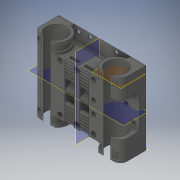
# Autodesk Inventor part: X-Carriage_back
Saved by Autodesk Inventor 2019 (Build 230136000, 136)
## iProperties
Created: 2019-09-14
Part Number: X-Carriage_back
Material: ABS-Kunststoff
Document SubType Name: Modeling
Designer: marc
Density: 1.06 g/cm^3
Appearance: Grau
Author: marc
## iProperties of the stored document X-Carriage_back_3D-Druck.ipt
Created: 2019-09-14
Part Number: X-Carriage_back_3D-Druck
Material: Generisch
Document SubType Name: Modeling
Designer: marc
Density: 1 g/cm^3
Appearance: Vorgabe
Author: marc
Autodesk Inventor part; units mm, degrees
ref_plane "YZ Plane" through (0, 0, 0) normal (1, 0, 0) x (0, 1, 0)
ref_plane "XZ Plane" through (0, 0, 0) normal (0, 1, 0) x (-1, 0, 0)
ref_plane "XY Plane" through (0, 0, 0) normal (0, 0, 1) x (1, 0, 0)
sketch "Skizze1" plane through (0, 0, 0) normal (0, 1, 0) x (-1, 0, 0)
  line L0 (0, 0) -> (65, 0)
  line L1 (65, 0) -> (65, 21.4)
  line L2 (65, 21.4) -> (0, 21.4)
  line L3 (0, 21.4) -> (0, 0)
  dimension "d0" = 65
  dimension "d1" = 21.4
  constraints: 8 end point, 2 parallel, 1 horizontal, 1 perpendicular
  measures "d0" distance of L2.end L1.end
  measures "d1" distance of L1.end L0.end
extrude "Extrusion1" add sketch "Skizze1" along normal blind 55
sketch "Skizze2" plane through (0, 0, 0) normal (0, -1, 0) x (1, 0, 0)
  line L0 (-65, 0) -> (-65, 21.4) projected
  line L1 (-65, 21.4) -> (0, 21.4) projected
  point P0 (0, 0)
  point P1 (-55, 9.4)
  point P2 (-10, 9.4)
  dimension "d4" = 10
  dimension "d5" = 45
  dimension "d6" = 12
  constraints: 1 horizontal alignment
  measures "d4" distance from line of L0 point (-55, 9.4)
  measures "d5" distance of point (-55, 9.4) point (-10, 9.4)
  measures "d6" distance from line of L1 point (-55, 9.4)
hole "Bohrung1" at (-55, 0, 9.4) at (-10, 0, 9.4) direction (0, 1, 0) diameter 15 end through all
sketch "Skizze7" plane through (0, 55, 0) normal (0, 1, 0) x (1, 0, 0)
  line L0 (-65, 0) -> (-65, -21.4) projected
  line L1 (0, -21.4) -> (0, 0) projected
  line L2 (-65, -21.4) -> (0, -21.4)
  line L3 (0, -21.4) -> (0, -16.4)
  line L4 (0, -16.4) -> (-65, -16.4)
  line L5 (-65, -16.4) -> (-65, -21.4)
  dimension "d49" = 5
  constraints: 8 end point, 2 parallel, 1 horizontal, 1 perpendicular, 1 point on line
  measures "d49" distance between parallel lines of L2 L4
extrude "Extrusion5" cut sketch "Skizze7" against normal up to next
sketch "Skizze8" plane through (0, 55, 0) normal (0, 1, 0) x (1, 0, 0)
  arc A0 (-52.3074, -16.4) -> (-57.6926, -16.4) centre (-55, -9.4) ccw projected
  line L0 (-45.7129, -11.4) -> (-19.2871, -11.4)
  arc A1 (-7.3074, -16.4) -> (-12.6926, -16.4) centre (-10, -9.4) ccw projected
  line L1 (0, 0) -> (-65, 0) projected
  line L2 (-52.3074, -16.4) -> (-12.6926, -16.4) projected
  arc A2 (-48.5774, -16.4) -> (-45.7129, -11.4) centre (-55, -9.4) ccw
  arc A3 (-19.2871, -11.4) -> (-16.4226, -16.4) centre (-10, -9.4) ccw
  dimension "d52" = 11.4
  dimension "d55" = 9.5
  dimension "d56" = 9.5
  constraints: 4 point on circle, 2 centre point, 2 coincident, 2 end point, 2 point on line, 1 horizontal
  measures "d52" distance between parallel lines of L1 L0
  measures "d55" radius of A3
  measures "d56" radius of A2
extrude "Extrusion6" cut sketch "Skizze8" against normal blind 7
ref_plane "Arbeitsebene3" through (0, 27.5, 0) normal (0, -1, 0) x (1, 0, 0)
mirror "Spiegeln3" about plane through (0, 27.5, 0) normal (0, -1, 0) of "Extrusion6"
ref_plane "Arbeitsebene4" through (-32.5, 0, 0) normal (-1, 0, 0) x (0, 0, 1)
sketch "Skizze9" plane through (0, 48, 0) normal (0, 1, 0) x (1, 0, 0)
  line L0 (-45.7129, -11.4) -> (-19.2871, -11.4) projected
  line L1 (-34.5, -11.4) -> (-41.5, -11.4)
  line L2 (-41.5, -11.4) -> (-41.5, -13.4)
  line L3 (-41.5, -13.4) -> (-34.5, -13.4)
  line L4 (-34.5, -13.4) -> (-34.5, -11.4)
  line L5 (-32.5, -19.68) -> (-32.5, 3.28) projected
  point P0 (0, 0)
  dimension "d59" = 7
  dimension "d60" = 2
  dimension "d61" = 2
  constraints: 8 end point, 2 parallel, 1 horizontal, 1 perpendicular, 1 point on line
  measures "d59" distance of L3.end L2.end
  measures "d60" distance of L2.end L1.end
  measures "d61" distance between parallel lines of L5 L4
extrude "Extrusion7" cut sketch "Skizze9" against normal blind 20
mirror "Spiegeln4" about plane through (-32.5, 0, 0) normal (-1, 0, 0) of "Extrusion7"
mirror "Spiegeln5" about plane through (0, 27.5, 0) normal (0, -1, 0) of "Extrusion7", "Spiegeln4"
sketch "Skizze10" plane through (-12.6926, 0, 16.4) normal (0, 0, 1) x (1, 0, 0)
  line L0 (-28.8074, 7) -> (-28.8074, 27) projected
  line L1 (-10.8074, 27) -> (-17.8074, 27) projected
  line L2 (-10.8074, 7) -> (-10.8074, 27) projected
  line L3 (-17.8074, 27) -> (-10.8074, 27)
  line L4 (-10.8074, 27) -> (-10.8074, 20)
  line L5 (-17.8074, 48) -> (-17.8074, 28) projected
  line L6 (-10.8074, 48) -> (-10.8074, 28) projected
  line L7 (-17.8074, 28) -> (-10.8074, 28)
  line L8 (-10.8074, 28) -> (-10.8074, 35)
  line L9 (-10.8074, 35) -> (-17.8074, 35)
  line L10 (-17.8074, 35) -> (-17.8074, 28)
  line L11 (-21.8074, 48) -> (-21.8074, 28) projected
  line L12 (-21.8074, 28) -> (-28.8074, 28)
  line L13 (-28.8074, 28) -> (-28.8074, 35)
  line L14 (-28.8074, 35) -> (-21.8074, 35)
  line L15 (-21.8074, 35) -> (-21.8074, 28)
  line L16 (-10.8074, 20) -> (-17.8074, 20)
  line L17 (-17.8074, 7) -> (-17.8074, 27) projected
  line L18 (-17.8074, 20) -> (-17.8074, 27)
  line L19 (-21.8074, 7) -> (-21.8074, 27) projected
  line L20 (-28.8074, 7) -> (-28.8074, 27) projected
  line L21 (-21.8074, 27) -> (-28.8074, 27)
  line L22 (-28.8074, 27) -> (-28.8074, 20)
  line L23 (-28.8074, 20) -> (-21.8074, 20)
  line L24 (-21.8074, 20) -> (-21.8074, 27)
  point P0 (12.6926, 0)
  dimension "d67" = 7
  dimension "d68" = 7
  dimension "d69" = 7
  constraints: 32 end point, 7 parallel, 7 point on line, 5 horizontal, 4 perpendicular, 1 vertical alignment
  measures "d67" distance between parallel lines of L7 L9
  measures "d68" distance of L3.end L4.end
  measures "d69" distance between parallel lines of L21 L23
extrude "Extrusion8" cut sketch "Skizze10" against normal up to next
fillet "Rundung3" radius 7 4 edges at (-38, 28, 11.4) (-27, 28, 11.4) (-38, 27, 11.4) (-27, 27, 11.4)
fillet "Rundung4" radius 1.5 8 edges at (-38, 35, 16.4) (-38, 35, 13.4) (-27, 35, 16.4) (-27, 35, 13.4) (-38, 20, 13.4) (-38, 20, 16.4) (-27, 20, 13.4) (-27, 20, 16.4)
sketch "Skizze11" plane through (-12.6926, 0, 16.4) normal (0, 0, 1) x (1, 0, 0)
  line L0 (-19.8074, -11) -> (-19.8074, 66) projected
  line L1 (-35.8848, 7) -> (-3.73, 7) projected
  point P0 (12.6926, 0)
  point P1 (-32.3074, 10)
  point P2 (-19.8074, 10)
  point P3 (-7.3074, 10)
  dimension "d71" = 12.5
  dimension "d72" = 12.5
  dimension "d73" = 3
  constraints: 2 horizontal alignment, 1 point on line
  measures "d71" distance from line of L0 point (-7.307, 10)
  measures "d72" distance from line of L0 point (-32.307, 10)
  measures "d73" distance from line of L1 point (-32.307, 10)
hole "Bohrung2" at (-45, 10, 16.4) at (-32.5, 10, 16.4) at (-20, 10, 16.4) direction (0, 0, -1) diameter 3.75 depth 8 tip angle 118
mirror "Spiegeln6" about plane through (0, 27.5, 0) normal (0, -1, 0) of "Bohrung2"
sketch "Skizze15" plane through (-12.6926, 0, 16.4) normal (0, 0, 1) x (1, 0, 0)
  line L0 (-28.8074, 7) -> (-21.8074, 7)
  line L1 (-21.8074, 7) -> (-21.8074, 18.5)
  line L2 (-21.8074, 18.5) -> (-28.8074, 18.5)
  line L3 (-28.8074, 18.5) -> (-28.8074, 7)
  line L4 (-35.8848, 7) -> (-3.73, 7) projected
  circle A0 centre (-32.3074, 10) radius 1.875 projected
  line L5 (-19.8074, -11) -> (-19.8074, 66) projected
  line L6 (-17.8074, 7) -> (-10.8074, 7)
  line L7 (-10.8074, 7) -> (-10.8074, 18.5)
  line L8 (-10.8074, 18.5) -> (-17.8074, 18.5)
  line L9 (-17.8074, 18.5) -> (-17.8074, 7)
  point P0 (12.6926, 0)
  constraints: 16 end point, 6 coincident, 4 parallel, 2 horizontal, 2 perpendicular, 2 point on line
extrude "Extrusion10" cut sketch "Skizze15" against normal blind 1.4 contours L3 L2 L1 L0 | L9 L8 L7 L4
sketch "Skizze16" plane through (-30.5, 7, 16.4) normal (1, 0, 0) x (0, 0, -1)
  line L0 (0, 0) -> (0, 11.5) projected
  line L1 (0, 11.5) -> (1.4, 11.5) projected
  line L2 (1.4, 0) -> (1.4, 11.5) projected
  line L3 (1.4, 0) -> (0, 0) projected
  arc A0 (0, 11.5) -> (0.4324, 10.9587) centre (0.555, 11.5) ccw
  arc A1 (0.4324, 10.9587) -> (1.024, 10.9328) centre (0.77, 11.9) ccw
  arc A2 (0.4324, 2.0413) -> (0.4324, 0.9587) centre (0.555, 1.5) ccw
  arc A3 (0.4324, 4.0413) -> (0.4324, 2.9587) centre (0.555, 3.5) ccw
  arc A4 (0.4324, 6.0413) -> (0.4324, 4.9587) centre (0.555, 5.5) ccw
  arc A5 (0.4324, 8.0413) -> (0.4324, 6.9587) centre (0.555, 7.5) ccw
  arc A6 (0.4324, 10.0413) -> (0.4324, 8.9587) centre (0.555, 9.5) ccw
  arc A7 (0.4324, 8.9587) -> (1.024, 8.9328) centre (0.77, 9.9) ccw
  arc A8 (1.024, 10.0672) -> (0.4324, 10.0413) centre (0.77, 9.1) ccw
  arc A9 (1.024, 8.0672) -> (0.4324, 8.0413) centre (0.77, 7.1) ccw
  arc A10 (0.4324, 6.9587) -> (1.024, 6.9328) centre (0.77, 7.9) ccw
  arc A11 (1.024, 2.0672) -> (0.4324, 2.0413) centre (0.77, 1.1) ccw
  arc A12 (0.4324, 4.9587) -> (1.024, 4.9328) centre (0.77, 5.9) ccw
  line L4 (1.024, 10.0672) -> (1.024, 10.9328)
  line L5 (1.024, 8.0672) -> (1.024, 8.9328)
  arc A13 (1.024, 6.0672) -> (0.4324, 6.0413) centre (0.77, 5.1) ccw
  line L6 (1.024, 6.0672) -> (1.024, 6.9328)
  line L7 (1.024, 4.0672) -> (1.024, 4.9328)
  line L8 (1.024, 0) -> (1.024, 0.9328)
  line L9 (1.024, 2.0672) -> (1.024, 2.9328)
  arc A14 (1.024, 4.0672) -> (0.4324, 4.0413) centre (0.77, 3.1) ccw
  arc A15 (0.4324, 2.9587) -> (1.024, 2.9328) centre (0.77, 3.9) ccw
  arc A16 (0.4324, 0.9587) -> (1.024, 0.9328) centre (0.77, 1.9) ccw
  point P0 (16.4, -7)
  point P1 (0.77, 11.1)
  dimension "d97" = 0.555
  dimension "d101" = 2
  dimension "d103" = 0.63
  dimension "d104" = 0.4
  dimension "d106" = 2
  dimension "d107" = 2
  dimension "d108" = 2
  dimension "d109" = 2
  dimension "d112" = 0.4
  dimension "d115" = 0.4
  dimension "d116" = 0.4
  dimension "d117" = 0.4
  dimension "d118" = 0.4
  dimension "d119" = 0.4
  dimension "d120" = 0.4
  dimension "d121" = 0.4
  dimension "d151" = 2
  dimension "d152" = 0.4
  dimension "d166" = 0.376
  dimension "d167" = 0.376
  dimension "d168" = 0.376
  dimension "d169" = 0.376
  dimension "d170" = 0.376
  dimension "d171" = 1
  dimension "d172" = 1
  dimension "d173" = 0.555
  dimension "d174" = 1
  dimension "d175" = 1
  dimension "d176" = 1
  dimension "d177" = 1
  dimension "d178" = 1
  dimension "d179" = 1
  dimension "d180" = 1
  dimension "d181" = 1
  dimension "d182" = 0.4
  dimension "d183" = 0.4
  dimension "d184" = 0.376
  constraints: 34 point on circle, 17 centre point, 16 coincident, 16 vertical alignment, 13 end point, 6 perpendicular, 6 tangent, 3 point on line
  measures "d97" distance from line of L0 point (0.555, 11.5)
  measures "d101" distance of point (0.555, 11.5) point (0.555, 9.5)
  measures "d103" distance from line of L2 point (0.77, 11.1)
  measures "d104" distance from line of L1 point (0.77, 11.1)
  measures "d106" distance of point (0.555, 9.5) point (0.555, 7.5)
  measures "d107" distance of point (0.555, 5.5) point (0.555, 7.5)
  measures "d108" distance of point (0.555, 3.5) point (0.555, 5.5)
  measures "d109" distance of point (0.555, 1.5) point (0.555, 3.5)
  measures "d112" vertical distance of point (0.555, 9.5) point (0.77, 9.9)
  measures "d115" vertical distance of point (0.555, 7.5) point (0.77, 7.1)
  measures "d116" vertical distance of point (0.555, 5.5) point (0.77, 5.9)
  measures "d117" vertical distance of point (0.555, 5.5) point (0.77, 5.1)
  measures "d118" vertical distance of point (0.555, 3.5) point (0.77, 3.9)
  measures "d119" vertical distance of point (0.555, 3.5) point (0.77, 3.1)
  measures "d120" vertical distance of point (0.555, 1.5) point (0.77, 1.9)
  measures "d121" vertical distance of point (0.555, 1.5) point (0.77, 1.1)
  measures "d151" diameter of A1
  measures "d152" distance from line of L1 A1.centre
  measures "d166" distance between parallel lines of L2 L5
  measures "d167" distance between parallel lines of L2 L6
  measures "d168" distance between parallel lines of L2 L7
  measures "d169" distance between parallel lines of L9 L2
  measures "d170" distance between parallel lines of L8 L2
  measures "d171" radius of A11
  measures "d172" radius of A16
  measures "d173" radius of A2
  measures "d174" radius of A15
  measures "d175" radius of A14
  measures "d176" radius of A12
  measures "d177" radius of A13
  measures "d178" radius of A10
  measures "d179" radius of A9
  measures "d180" radius of A7
  measures "d181" radius of A8
  measures "d182" vertical distance of point (0.555, 9.5) point (0.77, 9.1)
  measures "d183" vertical distance of point (0.555, 7.5) point (0.77, 7.9)
  measures "d184" distance between parallel lines of L2 L4
extrude "Extrusion11" add sketch "Skizze16" along normal up to next contours A2 A11 L9 A15 A3 A14 L7 A12 A4 A13 L6 A10 A5 A9 L5 A7 A6 A8 L4 A1 A0 L1 L2 L3 L8 A16
mirror "Spiegeln7" about plane through (-32.5, 0, 0) normal (-1, 0, 0) of "Extrusion11"
mirror "Spiegeln8" about plane through (0, 27.5, 0) normal (0, -1, 0) of "Extrusion11", "Spiegeln7", "Extrusion10"
sketch "Skizze18" plane through (0, 55, 0) normal (0, 1, 0) x (1, 0, 0)
  arc A0 (-52.3074, -16.4) -> (-57.6926, -16.4) centre (-55, -9.4) ccw projected
  arc A1 (-7.3074, -16.4) -> (-12.6926, -16.4) centre (-10, -9.4) ccw projected
  line L0 (-45.7129, -11.4) -> (-41.5, -11.4) projected
  arc A2 (-45.7129, -11.4) -> (-53.6252, 0) centre (-55, -9.4) ccw
  arc A3 (-11.3748, 0) -> (-19.2871, -11.4) centre (-10, -9.4) ccw
  line L1 (-19.2871, -11.4) -> (-45.7129, -11.4) projected
  line L2 (-45.7129, -11.4) -> (-19.2871, -11.4)
  line L3 (0, 0) -> (-65, 0) projected
  line L4 (-53.6252, 0) -> (-11.3748, 0)
  dimension "d190" = 45
  dimension "d192" = 19
  constraints: 4 end point, 4 point on circle, 3 point on line, 2 centre point, 2 coincident, 1 collinear
  measures "d190" distance of A0.centre A1.centre
  measures "d192" diameter of A3
extrude "Extrusion12" cut sketch "Skizze18" against normal up to surface (7 mm away)
mirror "Spiegeln9" about plane through (0, 27.5, 0) normal (0, -1, 0) of "Extrusion12"
sketch "Skizze19" plane through (-65, 0, 0) normal (0, 0, -1) x (-1, 0, 0)
  line L0 (13, 27.5) -> (-78, 27.5) projected
  line L1 (-65, 0) -> (-65, 55) projected
  point P0 (-45, 32)
  point P1 (-45, 23)
  point P2 (-55, 27.5)
  dimension "d195" = 10
  dimension "d196" = 20
  dimension "d197" = 20
  dimension "d198" = 4.5
  dimension "d200" = 4.5
  constraints: 1 point on line
  measures "d195" distance from line of L1 point (-55, 27.5)
  measures "d196" distance from line of L1 point (-45, 32)
  measures "d197" distance from line of L1 point (-45, 23)
  measures "d198" distance from line of L0 point (-45, 32)
  measures "d200" distance from line of L0 point (-45, 23)
hole "Bohrung3" at (-20, 32, 0) at (-20, 23, 0) at (-10, 27.5, 0) direction (0, 0, 1) diameter 3.2 end through all
ref_plane "Arbeitsebene6" through (0, 50.5, 0) normal (0, 1, 0) x (1, 0, 0)
sketch "Skizze21" plane through (0, 50.5, 0) normal (0, 1, 0) x (1, 0, 0)
  circle A0 centre (-10, -9.4) radius 9.75
  arc A1 (-7.3074, -16.4) -> (-12.6926, -16.4) centre (-10, -9.4) ccw projected
  circle A2 centre (-10, -9.4) radius 8
  point P0 (0, 0)
  dimension "d220" = 19.5
  dimension "d221" = 16
  constraints: 2 centre point, 1 coincident, 1 concentric
  measures "d220" diameter of A0
  measures "d221" diameter of A2
extrude "Extrusion13" cut sketch "Skizze21" along normal mid plane 4
mirror "Spiegeln10" about plane through (-32.5, 0, 0) normal (-1, 0, 0) of "Extrusion13"
mirror "Spiegeln11" about plane through (0, 27.5, 0) normal (0, -1, 0) of "Extrusion13", "Spiegeln10"
sketch "Skizze22" plane through (-65, 0, 0) normal (0, 0, -1) x (-1, 0, 0)
  circle A0 centre (-45, 23) radius 1.6 projected
  circle A1 centre (-45, 32) radius 1.6 projected
  circle A2 centre (-55, 27.5) radius 1.6 projected
  line L0 (-11.3748, 7) -> (-11.3748, 6.5) projected
  line L1 (-11.3748, 0) -> (0, 0) projected
  line L2 (0, 0) -> (0, 55) projected
  line L3 (-11.3748, 55) -> (0, 55) projected
  line L4 (-11.3748, 55) -> (-11.3748, 52.5) projected
  line L5 (-11.3748, 48) -> (-53.6252, 48) projected
  line L6 (-53.6252, 48) -> (-53.6252, 48.5) projected
  line L7 (-65, 55) -> (-53.6252, 55) projected
  line L8 (-65, 0) -> (-65, 55) projected
  line L9 (-65, 0) -> (-53.6252, 0) projected
  line L10 (-53.6252, 0) -> (-53.6252, 2.5) projected
  line L11 (-53.6252, 7) -> (-11.3748, 7) projected
  line L12 (-7.4111, 2.5) -> (-11.3748, 2.5) projected
  line L13 (-11.3748, 2.5) -> (-11.3748, 0) projected
  line L14 (-11.3748, 52.5) -> (-7.4111, 52.5) projected
  line L15 (-7.4111, 52.5) -> (-7.4111, 48.5) projected
  line L16 (-7.4111, 48.5) -> (-11.3748, 48.5) projected
  line L17 (-11.3748, 48.5) -> (-11.3748, 48) projected
  line L18 (-53.6252, 48.5) -> (-57.5889, 48.5) projected
  line L19 (-57.5889, 48.5) -> (-57.5889, 52.5) projected
  line L20 (-57.5889, 52.5) -> (-53.6252, 52.5) projected
  line L21 (-53.6252, 52.5) -> (-53.6252, 55) projected
  line L22 (-53.6252, 2.5) -> (-57.5889, 2.5) projected
  line L23 (-57.5889, 2.5) -> (-57.5889, 6.5) projected
  line L24 (-57.5889, 6.5) -> (-53.6252, 6.5) projected
  line L25 (-53.6252, 6.5) -> (-53.6252, 7) projected
  line L26 (-11.3748, 6.5) -> (-7.4111, 6.5) projected
  line L27 (-7.4111, 6.5) -> (-7.4111, 2.5) projected
extrude "Extrusion14" add sketch "Skizze22" along normal blind 3
sketch "Skizze23" plane through (-65, 0, -3) normal (0, 0, -1) x (-1, 0, 0)
  line L0 (0, 0) -> (0, 55) projected
  line L1 (0, 55) -> (-65, 55)
  line L2 (-65, 55) -> (-65, 0)
  line L3 (-65, 0) -> (0, 0)
  line L4 (0, 0) -> (0, 55)
  circle A0 centre (-45, 32) radius 1.6 projected
  circle A1 centre (-45, 23) radius 1.6 projected
  circle A2 centre (-55, 27.5) radius 1.6 projected
  constraints: 8 end point, 2 parallel, 1 horizontal, 1 perpendicular
extrude "Extrusion15" add sketch "Skizze23" along normal blind 1
sketch "Skizze24" plane through (-65, 0, -4) normal (0, 0, -1) x (-1, 0, 0)
  line L0 (0, 55) -> (-65, 55) projected
  line L1 (-32.5, 66) -> (-32.5, -11) projected
  point P0 (-65, 0)
  point P1 (-42.25, 52)
  point P2 (-22.75, 52)
  dimension "d228" = 3
  dimension "d229" = 3
  dimension "d230" = 19.5
  dimension "d231" = 9.75
  measures "d228" distance from line of L0 point (-42.25, 52)
  measures "d229" distance from line of L0 point (-22.75, 52)
  measures "d230" distance of point (-22.75, 52) point (-42.25, 52)
  measures "d231" distance from line of L1 point (-22.75, 52)
hole "Bohrung5" at (-22.75, 52, -4) at (-42.25, 52, -4) direction (0, 0, 1) diameter 3.1 end through all
mirror "Spiegeln12" [suppressed]
sketch "Skizze25" plane through (-7.3074, 55, 16.4) normal (0, 0, 1) x (1, 0, 0)
  line L0 (0, -55) -> (0, 0) projected
  line L1 (7.3074, -40) -> (0, -40)
  line L2 (0, -40) -> (0, -15)
  line L3 (0, -15) -> (7.3074, -15)
  line L4 (7.3074, -15) -> (7.3074, -40)
  line L5 (7.3074, -40) -> (0, -15) construction
  line L6 (0, -40) -> (7.3074, -15) construction
  line L7 (20.3074, -27.5) -> (-70.6926, -27.5) projected
  line L8 (7.3074, 0) -> (7.3074, -55) projected
  point P0 (3.6537, -27.5)
  point P1 (3.6537, -27.5)
  dimension "d239" = 25
  constraints: 12 end point, 3 midpoint, 3 point on line, 2 parallel, 1 horizontal, 1 perpendicular
  measures "d239" distance of L3.end L1.start
extrude "Extrusion16" cut sketch "Skizze25" against normal blind 14
sketch "Skizze26" plane through (-7.3074, 55, 2.4) normal (0, 0, 1) x (1, 0, 0)
  line L0 (20.3074, -27.5) -> (-70.6926, -27.5) projected
  line L1 (7.3074, -15) -> (7.3074, -40) projected
  point P0 (7.3074, -55)
  point P1 (3.3074, -36.7)
  point P2 (3.3074, -18.3)
  dimension "d242" = 18.4
  dimension "d243" = 9.2
  dimension "d244" = 4
  constraints: 1 vertical alignment
  measures "d242" distance of point (3.307, -18.3) point (3.307, -36.7)
  measures "d243" distance from line of L0 point (3.307, -18.3)
  measures "d244" distance from line of L1 point (3.307, -18.3)
hole "Bohrung6" at (-4, 18.3, 2.4) at (-4, 36.7, 2.4) direction (0, 0, -1) diameter 3.1 end through all
sketch "Skizze27" plane through (-65, 0, -4) normal (0, 0, -1) x (-1, 0, 0)
  line L0 (0, 55) -> (-65, 55) projected
  line L1 (-65, 55) -> (-65, 0) projected
  point P0 (-61, 51)
  point P1 (-51, 51)
  dimension "d252" = 4
  dimension "d253" = 4
  dimension "d254" = 4
  dimension "d255" = 10
  measures "d252" distance from line of L0 point (-51, 51)
  measures "d253" distance from line of L0 point (-61, 51)
  measures "d254" distance from line of L1 point (-61, 51)
  measures "d255" distance of point (-51, 51) point (-61, 51)
hole "Bohrung7" at (-14, 51, -4) direction (0, 0, 1) diameter 3.1 depth 2.5
hole "Bohrung8" at (-4, 51, -4) direction (0, 0, 1) diameter 3.75 depth 5
mirror "Spiegeln13" about plane through (0, 27.5, 0) normal (0, -1, 0) of "Bohrung7", "Bohrung8"
sketch "Skizze28" plane through (-65, 0, -4) normal (0, 0, -1) x (-1, 0, 0)
  point P0 (-65, 0)
mirror "Spiegeln14" about plane through (-32.5, 0, 0) normal (-1, 0, 0) of "Bohrung7", "Bohrung8", "Spiegeln13"
sketch "Skizze29" plane through (-65, 0, -4) normal (0, 0, -1) x (-1, 0, 0)
  line L0 (-58.0555, 36.7) -> (-59.5278, 34.15)
  line L1 (-59.5278, 34.15) -> (-62.4722, 34.15)
  line L2 (-62.4722, 34.15) -> (-63.9445, 36.7)
  line L3 (-63.9445, 36.7) -> (-62.4722, 39.25)
  line L4 (-62.4722, 39.25) -> (-59.5278, 39.25)
  line L5 (-59.5278, 39.25) -> (-58.0555, 36.7)
  line L6 (-58.0555, 18.3) -> (-59.5278, 15.75)
  line L7 (-59.5278, 15.75) -> (-62.4722, 15.75)
  line L8 (-62.4722, 15.75) -> (-63.9445, 18.3)
  line L9 (-63.9445, 18.3) -> (-62.4722, 20.85)
  line L10 (-62.4722, 20.85) -> (-59.5278, 20.85)
  line L11 (-59.5278, 20.85) -> (-58.0555, 18.3)
  line L12 (0, 55) -> (-65, 55) projected
  circle A0 centre (-61, 36.7) radius 1.55 projected
  circle A1 centre (-61, 18.3) radius 1.55 projected
  point P0 (-65, 0)
  dimension "d270" = 5.1
  dimension "d271" = 5.1
  constraints: 24 end point, 2 coincident, 2 parallel, 26 other
  measures "d270" distance between parallel lines of L7 L10
  measures "d271" distance between parallel lines of L4 L1
extrude "Extrusion17" cut sketch "Skizze29" against normal blind 2
fillet "Rundung6" radius 5 3 edges at (0, 47.5, 16.4) (0, 7.5, 16.4) (-65, 27.5, 16.4)
sketch "Skizze30" plane through (0, 48, 0) normal (0, 1, 0) x (1, 0, 0)
  line L0 (-34.5, -11.4) -> (-34.5, -13.4) projected
  line L1 (-34.5, -13.4) -> (-41.5, -13.4) projected
  line L2 (-41.5, -13.4) -> (-41.5, -11.4) projected
  line L3 (-34.5, -11.4) -> (-41.5, -11.4) projected
  arc A0 (-48.5774, -16.4) -> (-53.6252, 0) centre (-55, -9.4) ccw projected
  line L4 (-41.5, -16.4) -> (-48.5774, -16.4) projected
  line L5 (-41.5, -16.4) -> (-41.5, -15.376) projected
  line L6 (-34.5, -15.376) -> (-41.5, -15.376) projected
  line L7 (-34.5, -15.376) -> (-34.5, -16.4) projected
  line L8 (-30.5, -16.4) -> (-34.5, -16.4) projected
  line L9 (-30.5, -16.4) -> (-30.5, -15.376) projected
  line L10 (-30.5, -15.376) -> (-23.5, -15.376) projected
  line L11 (-23.5, -15.376) -> (-23.5, -16.4) projected
  line L12 (-16.4226, -16.4) -> (-23.5, -16.4) projected
  arc A1 (-11.3748, 0) -> (-16.4226, -16.4) centre (-10, -9.4) ccw projected
  line L13 (-11.3748, 0) -> (-11.3748, 3) projected
  line L14 (-53.6252, 3) -> (-11.3748, 3) projected
  line L15 (-53.6252, 0) -> (-53.6252, 3) projected
  line L16 (-23.5, -11.4) -> (-30.5, -11.4) projected
  line L17 (-23.5, -11.4) -> (-23.5, -13.4) projected
  line L18 (-23.5, -13.4) -> (-30.5, -13.4) projected
  line L19 (-30.5, -13.4) -> (-30.5, -11.4) projected
  point P0 (0, 0)
extrude "Extrusion18" cut sketch "Skizze30" against normal blind 0.75
sketch "Skizze31" plane through (0, 47.25, 0) normal (0, 1, 0) x (1, 0, 0)
  line L0 (-53.6252, 0) -> (-53.6252, 3) projected
  line L1 (-7.4111, 3) -> (-11.3748, 3) projected
  line L2 (-53.6252, 0) -> (-11.3748, 0)
  line L3 (-11.3748, 0) -> (-11.3748, 3)
  line L4 (-11.3748, 3) -> (-53.6252, 3)
  line L5 (-53.6252, 3) -> (-53.6252, 0)
  point P0 (0, 0)
  constraints: 8 end point, 2 parallel, 1 horizontal, 1 perpendicular
extrude "Extrusion19" cut sketch "Skizze31" against normal blind 2
chamfer "Fase1" distance 2 angle 45 1 edges at (-32.5, 47.25, 0)
fillet "Rundung7" radius 2 4 edges at (-65, 27.5, -4) (-32.5, 55, -4) (0, 27.5, -4) (-32.5, 0, -4)
equation "\"d69\" = d68"
equation "\"d115\" = d114"
equation "\"d116\" = d115"
equation "\"d117\" = d116"
equation "\"d118\" = d117"
equation "\"d119\" = d118"
equation "\"d120\" = d119"
equation "\"d121\" = d120"
equation "\"d54\" = d53"
equation "\"d113\" = d112"
equation "\"d114\" = d113"
equation "\"d53\" = 19"
